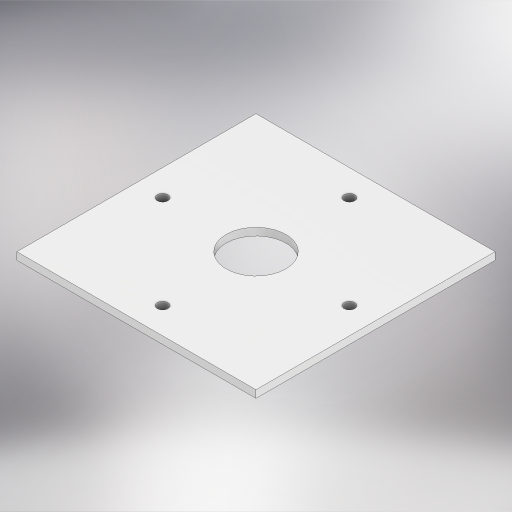
# Autodesk Inventor part: Top plate
Saved by Autodesk Inventor 2024 (Build 280153000, 153)
## iProperties
Created: 2023-10-09
Part Number: Top plate
Material: Acetal Resin, White
Document SubType Name: Modeling
Designer: byrne
Density: 1.425 g/cm^3
Appearance: Smooth - White
Author: byrne
Autodesk Inventor part; units mm, degrees
ref_plane "YZ Plane" through (0, 0, 0) normal (1, 0, 0) x (0, 1, 0)
ref_plane "XZ Plane" through (0, 0, 0) normal (0, 1, 0) x (-1, 0, 0)
ref_plane "XY Plane" through (0, 0, 0) normal (0, 0, 1) x (1, 0, 0)
sketch "Sketch1" plane through (0, 0, 0) normal (0, 1, 0) x (-1, 0, 0)
  line L0 (0, 0) -> (101.6, 0)
  line L1 (101.6, 0) -> (101.6, -101.6)
  line L2 (101.6, -101.6) -> (0, -101.6)
  line L3 (0, -101.6) -> (0, 0)
  circle A0 centre (90.4875, -50.8) radius 2.286
  circle A1 centre (50.8, -50.8) radius 12.7
  circle A2 centre (50.8, -90.4875) radius 2.286
  circle A3 centre (11.1125, -50.8) radius 2.286
  circle A4 centre (50.8, -11.1125) radius 2.286
  point P0 (101.6, -50.8)
  point P1 (50.8, -101.6)
  dimension "d0" = 101.6
  dimension "d1" = 101.6
  dimension "d2" = 4.572
  dimension "d3" = 11.1125
  dimension "d4" = 25.4
  dimension "d7" = 360
  constraints: 8 end point, 5 centre point, 2 horizontal alignment, 2 midpoint, 2 parallel, 1 coincident, 1 horizontal, 1 perpendicular, 1 vertical alignment, 9 other
  measures "d0" distance of L1.end L2.end
  measures "d1" distance of L0.end L1.end
  measures "d2" diameter of A0
  measures "d3" distance from line of L1 A0.centre
  measures "d4" diameter of A1
extrude "Extrusion1" add sketch "Sketch1" along normal blind 3.175
body "Solid1"
